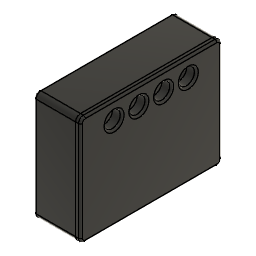
Display_Holder (Autodesk Fusion 360 design; units mm, degrees)
Autodesk Fusion 360 part; units mm, degrees
note: some values were not read from the file. Set by a fixed rule: which sketch regions a step uses.
sketch "Sketch1" plane through (0, 0, 0) normal (0, 0, 1) x (1, 0, 0)
  line L0 (13.5, -10.2) -> (-13.5, -10.2)
  line L1 (-13.5, -10.2) -> (-13.5, 10.2)
  line L2 (-13.5, 10.2) -> (13.5, 10.2)
  line L3 (13.5, 10.2) -> (13.5, -10.2)
  line L4 (13.5, -10.2) -> (-13.5, 10.2) construction
  line L5 (-13.5, -10.2) -> (13.5, 10.2) construction
  dimension "d1" = 27
  dimension "d2" = 20.4
  constraint horizontal L0
  constraint perpendicular L0 L1
  constraint parallel L0 L2
  constraint parallel L1 L3
  constraint coincident L4 origin
  constraint coincident L5 origin
  measures "d1" distance of L1.end L2.end
  measures "d2" distance of L0.end L1.end
extrude "Extrude1" add sketch "Sketch1" along normal blind 1 makes body 1
sketch "Sketch2" plane through (0, 0, 0) normal (0, 0, -1) x (1, 0, 0)
  line L0 (-13.5, -10.2) -> (13.5, -10.2)
  line L1 (13.5, -10.2) -> (13.5, 10.2)
  line L2 (13.5, 10.2) -> (-13.5, 10.2)
  line L3 (-13.5, 10.2) -> (-13.5, -10.2)
  circle A0 centre (7.6, 6.4) radius 0.8
  circle A1 centre (2.52, 6.4) radius 0.8
  circle A2 centre (-2.56, 6.4) radius 0.8
  circle A3 centre (-7.64, 6.4) radius 0.8
  circle A4 centre (10.5, 6.4) radius 0.8
  line L4 (-6.04, 4.8) -> (-9.24, 4.8)
  line L5 (-9.24, 4.8) -> (-9.24, 8)
  line L6 (-9.24, 8) -> (-6.04, 8)
  line L7 (-6.04, 8) -> (-6.04, 4.8)
  line L8 (-6.04, 4.8) -> (-9.24, 8) construction
  line L9 (-9.24, 4.8) -> (-6.04, 8) construction
  line L10 (-0.96, 4.8) -> (-4.16, 4.8)
  line L11 (-0.96, 8) -> (-0.96, 4.8)
  line L12 (-4.16, 8) -> (-0.96, 8)
  line L13 (-4.16, 4.8) -> (-4.16, 8)
  line L14 (4.12, 4.8) -> (0.92, 4.8)
  line L15 (4.12, 8) -> (4.12, 4.8)
  line L16 (0.92, 8) -> (4.12, 8)
  line L17 (0.92, 4.8) -> (0.92, 8)
  line L18 (9.2, 4.8) -> (6, 4.8)
  line L19 (9.2, 8) -> (9.2, 4.8)
  line L20 (6, 8) -> (9.2, 8)
  line L21 (6, 4.8) -> (6, 8)
  line L22 (12.1, 7.6) -> (8.9, 7.6)
  line L23 (8.9, 7.6) -> (8.9, 5.2)
  line L24 (8.9, 5.2) -> (12.1, 5.2)
  line L25 (12.1, 5.2) -> (12.1, 7.6)
  line L26 (12.1, 7.6) -> (8.9, 5.2) construction
  line L27 (8.9, 7.6) -> (12.1, 5.2) construction
  line L28 (8.9, 5.2) -> (12.1, 5.2)
  line L29 (12.1, 5.2) -> (12.1, 4.4)
  line L30 (12.1, 4.4) -> (8.9, 4.4)
  line L31 (8.9, 4.4) -> (8.9, 5.2)
  line L32 (9.2, 4.8) -> (12.4, 4.8)
  line L33 (12.4, 4.8) -> (12.4, 8)
  line L34 (12.4, 8) -> (9.2, 8)
  line L35 (9.2, 8) -> (9.2, 4.8)
  point P0 (-7.64, 6.4)
  point P1 (10.5, 6.4)
  dimension "d5" = 1.6
  dimension "d6" = 5.9
  dimension "d7" = 3.8
  dimension "d10" = -5.08
  dimension "d11" = 0
  dimension "d12" = 1.6
  dimension "d13" = 3.8
  dimension "d14" = 24
  dimension "d37" = 3.2
  dimension "d38" = 3.2
  dimension "d41" = -5.08
  dimension "d42" = 0
  dimension "d43" = 3.2
  dimension "d44" = 2.4
  dimension "d45" = 3.2
  dimension "d46" = 0.8
  dimension "d66" = 3.2
  dimension "d67" = 3.2
  constraint horizontal L4
  constraint perpendicular L4 L5
  constraint parallel L4 L6
  constraint parallel L5 L7
  constraint coincident L8 P0
  constraint coincident L9 P0
  constraint coincident P0 A3.centre
  constraint horizontal L22
  constraint perpendicular L22 L23
  constraint parallel L22 L24
  constraint parallel L23 L25
  constraint coincident L26 P1
  constraint coincident L27 P1
  constraint coincident P1 A4.centre
  constraint horizontal L28
  constraint vertical L29
  constraint horizontal L30
  constraint vertical L31
  constraint horizontal L32
  constraint vertical L33
  constraint horizontal L34
  constraint vertical L35
  measures "d5" diameter of A0
  measures "d6" distance of L1 A0.centre
  measures "d7" distance of L2 A0.centre
  measures "d12" diameter of A4
  measures "d13" distance of L2 P1
  measures "d14" distance of L3 P1
  measures "d37" distance of L5.end L6.end
  measures "d38" distance of L4.end L5.end
  measures "d43" distance of L23.end L24.end
  measures "d44" distance of L22.end L23.end
  measures "d45" distance of L23.end L24.end
  measures "d46" distance of L23.end L30.end
  measures "d66" distance of L18.start L32.end
  measures "d67" distance of L18.start L19.start
extrude "Extrude2" cut sketch "Sketch2" against normal blind 1 contours A0 | A1 | A2 | A3 | A4 | L4 L5 L6 L7 | L10 L11 L12 L13 | L14 L15 L16 L17 | L18 L19 L24 L28 L31 L35 | L19 L24 L28 L29 L32 L35 | L18 L19 L20 L21 L22 L23 L31 L35 | L19 L22 L23 L24 L28 L35 | L19 L22 L24 L25 L28 L35 | L19 L22 L25 L29 L32 L33 L34 L35 bodies 1
sketch "Sketch3" plane through (0, 0, 0) normal (0, 0, -1) x (1, 0, 0)
  line L0 (4.12, 8) -> (4.12, 4.8)
  line L1 (4.12, 4.8) -> (0.92, 4.8)
  line L2 (0.92, 4.8) -> (0.92, 8)
  line L3 (0.92, 8) -> (4.12, 8)
  line L4 (-0.96, 8) -> (-0.96, 4.8)
  line L5 (-0.96, 4.8) -> (-4.16, 4.8)
  line L6 (-4.16, 4.8) -> (-4.16, 8)
  line L7 (-4.16, 8) -> (-0.96, 8)
  line L8 (12.4, 8) -> (12.4, 4.8)
  line L9 (12.4, 4.8) -> (6, 4.8)
  line L10 (6, 4.8) -> (6, 8)
  line L11 (6, 8) -> (12.4, 8)
  line L12 (-9.24, 4.8) -> (-9.24, 8)
  line L13 (-9.24, 8) -> (-6.04, 8)
  line L14 (-6.04, 8) -> (-6.04, 4.8)
  line L15 (-6.04, 4.8) -> (-9.24, 4.8)
  line L16 (-13.5, -10.2) -> (13.5, -10.2)
  line L17 (13.5, -10.2) -> (13.5, 10.2)
  line L18 (13.5, 10.2) -> (-13.5, 10.2)
  line L19 (-13.5, 10.2) -> (-13.5, -10.2)
  line L20 (14.5, 11.2) -> (-14.5, 11.2)
  line L21 (-14.5, 11.2) -> (-14.5, -11.2)
  line L22 (-14.5, -11.2) -> (14.5, -11.2)
  line L23 (14.5, -11.2) -> (14.5, 11.2)
  dimension "d68" = 1
extrude "Extrude3" add sketch "Sketch3" against normal blind 1 contours L20 L21 L22 L23 bodies 1
extrude "Extrude4" add sketch "Sketch3" along normal blind 7.5 contours L20 L21 L22 L23 bodies 1
sketch "Sketch4" plane through (0, 0, 0) normal (0, 0, -1) x (1, 0, 0)
  line L0 (13.5, -10.2) -> (-13.5, -10.2)
  line L1 (-13.5, -10.2) -> (-13.5, -4.2)
  line L2 (-13.5, -4.2) -> (13.5, -4.2)
  line L3 (13.5, -4.2) -> (13.5, -10.2)
  line L4 (-0.96, 8) -> (-0.96, 4.8)
  line L5 (-0.96, 4.8) -> (-4.16, 4.8)
  line L6 (-4.16, 4.8) -> (-4.16, 8)
  line L7 (-4.16, 8) -> (-0.96, 8)
  line L8 (-9.24, 4.8) -> (-9.24, 8)
  line L9 (-9.24, 8) -> (-6.04, 8)
  line L10 (-6.04, 8) -> (-6.04, 4.8)
  line L11 (-6.04, 4.8) -> (-9.24, 4.8)
  line L12 (4.12, 8) -> (4.12, 4.8)
  line L13 (4.12, 4.8) -> (0.92, 4.8)
  line L14 (0.92, 4.8) -> (0.92, 8)
  line L15 (0.92, 8) -> (4.12, 8)
  line L16 (12.4, 4.8) -> (6, 4.8)
  line L17 (6, 4.8) -> (6, 8)
  line L18 (12.4, 8) -> (12.4, 4.8)
  line L19 (6, 8) -> (12.4, 8)
  line L20 (-13.5, -10.2) -> (13.5, -10.2)
  line L21 (13.5, -10.2) -> (13.5, 10.2)
  line L22 (13.5, 10.2) -> (-13.5, 10.2)
  line L23 (-13.5, 10.2) -> (-13.5, -10.2)
  dimension "d22" = 6
  constraint horizontal L0
  constraint vertical L1
  constraint horizontal L2
  constraint vertical L3
  constraint coincident L1.end L23
  measures "d22" distance of L0.start L2.end
extrude "Extrude5" add sketch "Sketch4" along normal blind 0.6 contours L0 L1 L2 L3 L20 L21 L23 bodies 1
sketch "Sketch5" plane through (0, 0, -7.5) normal (0, 0, -1) x (1, 0, 0)
  line L0 (-13.5, -10.2) -> (-13.5, 10.2)
  line L1 (-13.5, 10.2) -> (13.5, 10.2)
  line L2 (13.5, 10.2) -> (13.5, -10.2)
  line L3 (13.5, -10.2) -> (-13.5, -10.2)
  line L4 (14.5, -11.2) -> (14.5, 11.2)
  line L5 (14.5, 11.2) -> (-14.5, 11.2)
  line L6 (-14.5, 11.2) -> (-14.5, -11.2)
  line L7 (-14.5, -11.2) -> (14.5, -11.2)
extrude "Extrude6" add sketch "Sketch5" against normal blind 1 separate body contours L0 L1 L2 L3 makes body 2
extrude "Extrude7" add sketch "Sketch5" along normal blind 1 contours L0 L1 L2 L3 | L4 L5 L6 L7 bodies 2
sketch "Sketch6" plane through (0, 0, -8.5) normal (0, 0, -1) x (1, 0, 0)
  circle A0 centre (7.6, 7.7) radius 0.8
  line L0 (7.6, 7.7) -> (7.6, -11.2)
  circle A1 centre (7.6, -7.5) radius 1.65
  circle A2 centre (2.52, -7.5) radius 1.65
  circle A3 centre (-2.56, -7.5) radius 1.65
  circle A4 centre (-7.64, -7.5) radius 1.65
  line L1 (-14.5, -11.2) -> (14.5, -11.2)
  line L2 (14.5, -11.2) -> (14.5, 11.2)
  line L3 (14.5, 11.2) -> (-14.5, 11.2)
  line L4 (-14.5, 11.2) -> (-14.5, -11.2)
  dimension "d29" = 3.3
  dimension "d33" = -5.08
  dimension "d34" = 0
  dimension "d51" = 1.6
  constraint coincident A0.centre L0.start
  constraint coincident L0 A1.centre
  measures "d29" diameter of A1
  measures "d51" diameter of A0
extrude "Extrude8" cut sketch "Sketch6" against normal blind 2 contours L0 A1 | L0 A1 | A2 | A3 | A4 bodies 2
fillet "Fillet1" radius 0.4 16 edges at (-6.04, -4.8, 0.5) (-9.24, -4.8, 0.5) (-9.24, -8, 0.5) (-6.04, -8, 0.5) (-4.16, -4.8, 0.5) (-0.96, -4.8, 0.5) (-0.96, -8, 0.5) (-4.16, -8, 0.5) (0.92, -4.8, 0.5) (4.12, -4.8, 0.5) (0.92, -8, 0.5) (4.12, -8, 0.5) (6, -4.8, 0.5) (6, -8, 0.5) (12.4, -4.8, 0.5) (12.4, -8, 0.5) on bodies 1
move_body "Move1" bodies 1 2 to x (1, 0, 0) y (0, -1, 0) z (0, 0, -1) at (0, -22.4, -15)
move_body "Move2" bodies 1 2 to x (1, 0, 0) y (0, 1, 0) z (0, 0, 1) at (0, 22.4, 16)
move_body "Move3" bodies 1 2 to x (0, -1, 0) y (1, 0, 0) z (0, 0, 1) at (0, 0, 0)
move_body "Move4" bodies 1 2 to x (0, 0, -1) y (0, 1, 0) z (1, 0, 0) at (0, 0, 0)
move_body "Move5" bodies 1 2 to x (1, 0, 0) y (0, 1, 0) z (0, 0, 1) at (-4.75, 0, 11.2)
fillet "Fillet6" radius 1 8 edges at (-0.5, -14.5, 22.4) (-0.5, 14.5, 22.4) (-0.5, -14.5, 0) (-0.5, 14.5, 0) (4.25, 14.5, 0) (4.25, 14.5, 22.4) (4.25, -14.5, 22.4) (4.25, -14.5, 0) on bodies 1 2
fillet "Fillet6" radius 0.5 4 edges at (0.3, -13.5, 21.4) (0, -13.5, 1) (0, 13.5, 1) (0.3, 13.5, 21.4) on bodies 1 2
fillet "Fillet7" radius 0.4 2 faces at (-4.75, -0.4168, 17.0646) (4.75, -0.7176, 5.6971) on bodies 1 2
equation "d10 = ( -2 * 2.54 ) * 1 mm"
equation "d13 = d7"
equation "d33 = ( -2.54 * 2 ) * 1 mm"
equation "d41 = ( -2 * 2.54 ) * 1 mm"
named bodies: "Holder", "Cap"
